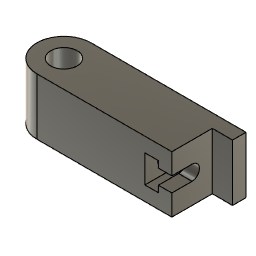
deltaz_assembly (Autodesk Fusion 360 archive; units mm, degrees)
design "forearm_educational"
Autodesk Fusion 360 part; units mm, degrees
sketch "Sketch1" plane through (0, 0, 0) normal (0, 0, 1) x (1, 0, 0)
  circle A0 centre (0, 0) radius 1.5
  line L0 (0, 6) -> (30, 6)
  line L1 (0, -6) -> (30, -6)
  arc A1 (0, 6) -> (0, -6) centre (0, 0) ccw
  line L2 (30, 6) -> (30, -6)
  dimension "d1" = 3
  dimension "d3" = 12
  dimension "d4" = 30
  constraint coincident A0.centre A1.centre
  constraint vertical L2
  constraint equal L0 L1
  constraint parallel L0 L1
  constraint horizontal L1
  constraint tangent L0 A1
  measures "d1" diameter of A0
  measures "d3" distance of L0.end L1.end
  measures "d4" distance of A0.centre L2
extrude "Extrude1" add sketch "Sketch1" along normal blind 12.6 makes body 1
sketch "Sketch2" plane through (30, 0, 0) normal (1, 0, 0) x (0, 1, 0)
  line L0 (-6, 0) -> (6, 0)
  line L1 (6, 0) -> (6, 12.6)
  line L2 (6, 12.6) -> (-6, 12.6)
  line L3 (-6, 12.6) -> (-6, 0)
  line L4 (6, 12.6) -> (3, 12.6)
  line L5 (3, 12.6) -> (3, 0)
  line L6 (3, 0) -> (6, 0)
  line L7 (6, 0) -> (6, 12.6)
  dimension "d7" = 3
  constraint horizontal L4
  constraint vertical L5
  constraint horizontal L6
  constraint vertical L7
  constraint coincident L0 L5.end
  constraint coincident L1.end L2.start
  measures "d7" distance of L5 L7
extrude "Extrude2" add sketch "Sketch2" along normal blind 4.5 contours L0 L1 L2 L4 L5 L6 L7 bodies 1
ref_plane "WorkPlane1" through (14.25, 0, 6.3) normal (0, 0, 1) x (1, 0, 0)
ref_plane "WorkPlane2" through (15, 0, 6.3) normal (0, -1, 0) x (1, 0, 0)
sketch "Sketch3" plane through (0, -6, 0) normal (0, -1, 0) x (1, 0, 0)
  line L0 (0, 0) -> (30, 0)
  line L1 (30, 0) -> (30, 12.6)
  line L2 (30, 12.6) -> (0, 12.6)
  line L3 (0, 12.6) -> (0, 0)
  line L4 (13, 10.8) -> (24, 10.8)
  line L5 (24, 10.8) -> (24, 1.8)
  line L6 (24, 1.8) -> (13, 1.8)
  line L7 (13, 1.8) -> (13, 10.8)
  point P0 (30, 6.3)
  point P1 (24, 6.3)
  dimension "d15" = 9
  dimension "d16" = 11
  dimension "d17" = 6
  constraint horizontal L4
  constraint vertical L5
  constraint horizontal L6
  constraint vertical L7
  constraint midpoint L5 P1
  constraint horizontal P0 P1
  constraint midpoint L1 P0
  measures "d15" distance of L4.start L6.end
  measures "d16" distance of L5.end L6.end
  measures "d17" distance of L1 L5
sketch "Sketch6" plane through (0, -6, 0) normal (0, -1, 0) x (1, 0, 0)
  line L0 (0, 0) -> (30, 0)
  line L1 (30, 0) -> (30, 12.6)
  line L2 (30, 12.6) -> (0, 12.6)
  line L3 (0, 12.6) -> (0, 0)
  line L4 (24, 9.4) -> (27, 9.4)
  line L5 (27, 3.2) -> (24, 3.2)
  line L6 (24, 3.2) -> (24, 9.4)
  line L7 (27, 4.65) -> (30, 4.65)
  line L8 (30, 4.65) -> (30, 7.95)
  line L9 (30, 7.95) -> (27, 7.95)
  line L10 (27, 9.4) -> (27, 7.95)
  line L11 (27, 4.65) -> (27, 3.2)
  dimension "d28" = 3
  dimension "d29" = 3
  dimension "d30" = 3.3
  dimension "d39" = 6.2
  constraint horizontal L4
  constraint vertical L10
  constraint horizontal L5
  constraint vertical L6
  constraint horizontal L7
  constraint vertical L8
  constraint horizontal L9
  constraint coincident L1 L8.end
  constraint collinear L10 L11
  constraint midpoint L1 L8
  constraint equal L10 L11
  measures "d28" distance of L4.start L4.end
  measures "d29" distance of L1 L11
  measures "d30" distance of L7 L9
  measures "d39" distance of L4.start L5.end
ref_plane "WorkPlane3" through (15, -1.5, 6.3) normal (0, -1, 0) x (1, 0, 0)
extrude "Extrude6" cut sketch "Sketch6" against normal up to surface (4.5 mm away) contours L1 L4 L5 L6 L7 L8 L9 L10 L11 bodies 1
sketch "Sketch7" plane through (30, 0, 0) normal (1, 0, 0) x (0, 1, 0)
  line L0 (-6, 7.95) -> (-1.5, 7.95)
  line L1 (-1.5, 7.95) -> (-1.5, 4.65)
  line L2 (-1.5, 4.65) -> (-6, 4.65)
  line L3 (-6, 4.65) -> (-6, 0)
  line L4 (-6, 0) -> (3, 0)
  line L5 (3, 0) -> (3, 12.6)
  line L6 (3, 12.6) -> (-6, 12.6)
  line L7 (-6, 12.6) -> (-6, 7.95)
  circle A0 centre (-1.5, 6.3) radius 1.65
  constraint midpoint L1 A0.centre
  constraint tangent L0 A0
extrude "Extrude7" cut sketch "Sketch7" against normal blind 7 contours L1 A0 | L1 A0 bodies 1
sketch "Sketch8" plane through (24, 0, 0) normal (1, 0, 0) x (0, 1, 0)
  arc A0 (-1.5, 7.95) -> (-1.5, 4.65) centre (-1.5, 6.3) ccw
  line L0 (-1.5, 7.95) -> (-1.5, 9.4)
  line L1 (-1.5, 9.4) -> (-6, 9.4)
  line L2 (-6, 9.4) -> (-6, 3.2)
  line L3 (-6, 3.2) -> (-1.5, 3.2)
  line L4 (-1.5, 3.2) -> (-1.5, 4.65)
  line L5 (-3.2898, 9.4) -> (0.2898, 9.4)
  line L6 (0.2898, 9.4) -> (2.0796, 6.3)
  line L7 (2.0796, 6.3) -> (0.2898, 3.2)
  line L8 (0.2898, 3.2) -> (-3.2898, 3.2)
  line L9 (-3.2898, 3.2) -> (-5.0796, 6.3)
  line L10 (-5.0796, 6.3) -> (-3.2898, 9.4)
  line L11 (-1.5, 9.4) -> (-1.5, 3.2) construction
  point P0 (-1.5, 9.4)
  point P1 (-1.5, 3.2)
  point P2 (-1.5, 6.3)
  dimension "d36" = 120
  constraint horizontal L5
  constraint parallel L5 L8
  constraint coincident L5 P0
  constraint midpoint L8 P1
  constraint coincident P0 L0.end
  constraint coincident P1 L3.end
  constraint midpoint L11 P2
  constraint equal L5 L6
  constraint equal L6 L7
  constraint equal L7 L8
  constraint equal L8 L9
  constraint equal L9 L10
  constraint vertical L11
  constraint midpoint L5 P0
  constraint coincident P2 A0.centre
  constraint collinear L1 L5
  measures "d36" angle of L5 L6
extrude "Extrude8" cut sketch "Sketch8" along normal up to surface (3 mm away) contours A0 L0 L4 L5 L6 L7 L8 | A0 L0 L1 L3 L4 L5 L8 L9 L10 bodies 1
sketch "Sketch10" plane through (0, 0, 12.6) normal (0, 0, 1) x (-1, 0, 0)
  circle A0 centre (0, 0) radius 1.5
  arc A1 (0, -6) -> (0, 6) centre (0, 0) ccw
  line L0 (0, 6) -> (-30, 6)
  line L1 (-30, 6) -> (-30, -3)
  line L2 (-30, -3) -> (-34.5, -3)
  line L3 (-34.5, -3) -> (-34.5, -6)
  line L4 (-34.5, -6) -> (0, -6)
  circle A2 centre (0, 0) radius 2.945
  dimension "d40" = 5.89
  constraint concentric A0 A2
  measures "d40" diameter of A2
extrude "Extrude9" cut sketch "Sketch10" against normal blind 7.1 contours A2 bodies 1
sketch "Sketch11" plane through (0, 0, 0) normal (0, 0, -1) x (1, 0, 0)
  circle A0 centre (0, 0) radius 1.5
  arc A1 (0, 6) -> (0, -6) centre (0, 0) ccw
  line L0 (0, -6) -> (34.5, -6)
  line L1 (34.5, -6) -> (34.5, -3)
  line L2 (34.5, -3) -> (30, -3)
  line L3 (30, -3) -> (30, 6)
  line L4 (30, 6) -> (0, 6)
  circle A2 centre (0, 0) radius 2.4
  dimension "d43" = 4.8
  constraint concentric A0 A2
  measures "d43" diameter of A2
extrude "Extrude10" cut sketch "Sketch11" against normal blind 3.5 contours A2 bodies 1
copy_body "Body->Comp1" bodies 1 removing the originals makes body 2 in component "Component"
sketch "Sketch12" plane through (0, -6, 0) normal (0, -1, 0) x (1, 0, 0)
  line L0 (27, 7.95) -> (30, 7.95)
  line L1 (30, 7.95) -> (30, 12.6)
  line L2 (30, 12.6) -> (0, 12.6)
  line L3 (0, 12.6) -> (0, 0)
  line L4 (0, 0) -> (30, 0)
  line L5 (30, 0) -> (30, 4.65)
  line L6 (30, 4.65) -> (27, 4.65)
  line L7 (27, 4.65) -> (27, 3.2)
  line L8 (27, 3.2) -> (24.6, 3.2)
  line L9 (24.6, 3.2) -> (24.6, 9.4)
  line L10 (24.6, 9.4) -> (27, 9.4)
  line L11 (27, 9.4) -> (27, 7.95)
  line L12 (-8, 12.6) -> (20, 12.6)
  line L13 (20, 12.6) -> (20, 0)
  line L14 (20, 0) -> (-8, 0)
  line L15 (-8, 0) -> (-8, 12.6)
  constraint horizontal L12
  constraint vertical L13
  constraint horizontal L14
  constraint vertical L15
  constraint coincident L4 L13.end
  constraint collinear L2 L12
extrude "Extrude11" [suppressed]
component "Component" placed x (1, 0, 0) y (0, 1, 0) z (0, 0, 1) at (0, 0, 0)
